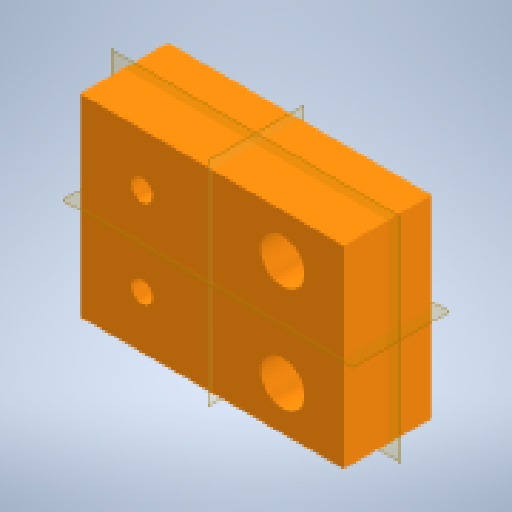
# Autodesk Inventor part: suporte_microswitch_001
Saved by Autodesk Inventor 2026 (Build 300175000, 175)
## iProperties
Created: 2025-11-26
Part Number: suporte_microswitch_001
Material: ABS Plastic
Document SubType Name: Modeling
Designer: Carlos Dias
Density: 1.06 g/cm^3
Appearance: Orange
Author: Carlos Dias
Autodesk Inventor part; units mm, degrees
sketch "Sketch1" plane through (0, 0, 0) normal (0, 0, 1) x (1, 0, 0)
  line L0 (-15, 11) -> (15, 11)
  line L1 (15, 11) -> (15, -11)
  line L2 (15, -11) -> (-15, -11)
  line L3 (-15, -11) -> (-15, 11)
  line L4 (-15, 11) -> (15, -11) construction
  line L5 (15, 11) -> (-15, -11) construction
  circle A0 centre (-8, 5) radius 1.2
  circle A1 centre (-8, -5) radius 1.2
  line L6 (-8, 5) -> (-8, -5) construction
  circle A2 centre (8, 6) radius 2.5
  circle A3 centre (8, -6) radius 2.5
  line L7 (8, 6) -> (8, -6) construction
  point P0 (0, 0)
  point P1 (0, 0)
  point P2 (-8, 0)
  point P3 (8, 0)
  dimension "d2" = 30
  dimension "d3" = 22
  dimension "d6" = 2.4
  dimension "d7" = 10
  dimension "d8" = 8
  dimension "d11" = 5
  dimension "d12" = 8
  dimension "d13" = 12
  constraints: 16 end point, 5 coincident, 4 centre point, 4 midpoint, 2 equal radius, 2 horizontal alignment, 2 parallel, 2 vertical, 1 horizontal, 1 perpendicular, 1 vertical alignment
  measures "d2" distance of L0.start L0.end
  measures "d3" distance of L0.end L1.end
  measures "d6" diameter of A0
  measures "d7" distance of A1.centre A0.centre
  measures "d8" distance from line of point (0, 0) L6
  measures "d11" diameter of A2
  measures "d12" distance of point (0, 0) point (8, 0)
  measures "d13" distance of L7.start L7.end
extrude "Extrusion3" add sketch "Sketch1" along normal mid plane 9
body "Solid3"
